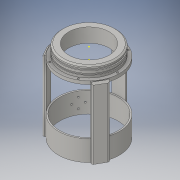
# Autodesk Inventor part: O ring fitting with motor mount
Saved by Autodesk Inventor 2016 (Build 200138000, 138)
## iProperties
Created: 2017-01-20
Part Number: O ring fitting with motor mount
Material: Generic
Document SubType Name: Modeling
Designer: Student
Density: 1 g/cm^3
Appearance: Default
Author: Student
Autodesk Inventor part; units mm, degrees
ref_plane "YZ Plane" through (0, 0, 0) normal (1, 0, 0) x (0, 1, 0)
ref_plane "XZ Plane" through (0, 0, 0) normal (0, 1, 0) x (-1, 0, 0)
ref_plane "XY Plane" through (0, 0, 0) normal (0, 0, 1) x (1, 0, 0)
sketch "Sketch1" plane through (0, 0, 0) normal (0, 1, 0) x (-1, 0, 0)
  circle A0 centre (0, 0) radius 50.8
  dimension "d0" = 101.6
  constraints: 1 centre point, 1 coincident
  measures "d0" diameter of A0
extrude "Extrusion1" add sketch "Sketch1" along normal blind 7.62
sketch "Sketch2" plane through (0, 7.62, 0) normal (0, 1, 0) x (1, 0, 0)
  circle A0 centre (0, 0) radius 49.2125
  circle A1 centre (0, 0) radius 50.8
  dimension "d3" = 98.425
  constraints: 2 centre point, 2 coincident
  measures "d3" diameter of A0
extrude "Extrusion2" cut sketch "Sketch2" against normal blind 3.175
sketch "Sketch3" plane through (0, 7.62, 0) normal (0, 1, 0) x (1, 0, 0)
  circle A0 centre (0, 0) radius 50.9584
  constraints: 1 centre point, 1 coincident
extrude "Extrusion3" add sketch "Sketch3" along normal blind 7.62
sketch "Sketch4" plane through (0, 15.24, 0) normal (0, 1, 0) x (1, 0, 0)
  point P0 (0, 0)
sketch "Sketch5" plane through (0, 15.24, 0) normal (0, 1, 0) x (1, 0, 0)
  circle A0 centre (0, 0) radius 49.2125
  circle A1 centre (0, 0) radius 50.9584
  dimension "d8" = 98.425
  constraints: 2 centre point, 2 coincident
  measures "d8" diameter of A0
extrude "Extrusion4" cut sketch "Sketch5" against normal blind 3.175
sketch "Sketch6" plane through (0, 15.24, 0) normal (0, 1, 0) x (1, 0, 0)
  circle A0 centre (0, 0) radius 50.8
  dimension "d11" = 101.6
  constraints: 1 centre point, 1 coincident
  measures "d11" diameter of A0
extrude "Extrusion5" add sketch "Sketch6" along normal blind 5.08
sketch "Sketch7" plane through (0, 0, 0) normal (0, -1, 0) x (1, 0, 0)
  circle A0 centre (0, 0) radius 57.15
  dimension "d14" = 114.3
  constraints: 1 centre point, 1 coincident
  measures "d14" diameter of A0
extrude "Extrusion6" add sketch "Sketch7" along normal blind 6.096
chamfer "Chamfer1" distance 2.54 angle 45 1 edges at (-50.8, 20.32, 0)
sketch "Sketch8" plane through (0, -6.096, 0) normal (0, -1, 0) x (1, 0, 0)
  circle A0 centre (0, 0) radius 50.8
  circle A1 centre (53.975, 0) radius 1.7526
  circle A2 centre (26.9875, 46.7437) radius 1.7526
  circle A3 centre (-26.9875, 46.7437) radius 1.7526
  circle A4 centre (-53.975, 0) radius 1.7526
  circle A5 centre (-26.9875, -46.7437) radius 1.7526
  circle A6 centre (26.9875, -46.7437) radius 1.7526
  dimension "d20" = 3.5052
  dimension "d21" = 53.975
  dimension "d24" = 360
  constraints: 7 centre point, 1 coincident, 13 other
  measures "d20" diameter of A1
  measures "d21" distance of A0.centre A1.centre
extrude "Extrusion7" cut sketch "Sketch8" against normal blind 6.096 contours A1 | A2 | A3 | A4 | A5 | A6
sketch "Sketch9" plane through (0, -6.096, 0) normal (0, -1, 0) x (1, 0, 0)
  circle A0 centre (0, 0) radius 12.7
  circle A1 centre (0, 0) radius 1.27
  dimension "d28" = 25.4
  dimension "d29" = 2.54
  constraints: 2 centre point, 2 coincident
  measures "d28" diameter of A0
  measures "d29" diameter of A1
extrude "Extrusion8" cut sketch "Sketch9" against normal blind 127 contours A1
sketch "Sketch10" plane through (0, -6.096, 0) normal (0, -1, 0) x (1, 0, 0)
  circle A0 centre (0, 0) radius 1.27 projected
  circle A1 centre (0, 0) radius 38.1
  dimension "d33" = 76.2
  constraints: 1 centre point, 1 coincident
  measures "d33" diameter of A1
extrude "Extrusion9" cut sketch "Sketch10" against normal blind 9.525
sketch "Sketch11" plane through (0, 3.429, 0) normal (0, -1, 0) x (1, 0, 0)
  circle A0 centre (0, 0) radius 12.7
  circle A1 centre (0, 0) radius 1.27
  dimension "d36" = 25.4
  constraints: 2 centre point, 2 coincident
  measures "d36" diameter of A0
extrude "Extrusion10" add sketch "Sketch11" along normal blind 9.525
sketch "Sketch12" plane through (0, 20.32, 0) normal (0, 1, 0) x (1, 0, 0)
  circle A0 centre (0, 0) radius 1.27 projected
  circle A1 centre (0, 0) radius 38.1
  constraints: 1 centre point, 1 coincident
extrude "Extrusion11" cut sketch "Sketch12" against normal blind 508
sketch "Sketch13" plane through (0, -6.096, 0) normal (0, -1, 0) x (1, 0, 0)
  point P0 (0, 0)
sketch "Sketch14" plane through (0, -6.096, 0) normal (0, -1, 0) x (1, 0, 0)
  line L0 (0, -60.96) -> (12.7, -60.96)
  line L1 (0, -60.96) -> (-12.7, -60.96)
  circle A0 centre (0, 0) radius 57.15 projected
  arc A1 (-12.7, -55.721) -> (12.7, -55.721) centre (0, 0) ccw
  line L2 (12.7, -60.96) -> (12.7, -55.721)
  line L3 (-12.7, -60.96) -> (-12.7, -55.721)
  line L4 (52.7929, 30.48) -> (59.1429, 19.4815)
  line L5 (52.7929, 30.48) -> (46.4429, 41.4785)
  line L6 (46.4429, 41.4785) -> (41.9058, 38.859)
  arc A2 (54.6058, 16.862) -> (41.9058, 38.859) centre (0, 0) ccw
  line L7 (59.1429, 19.4815) -> (54.6058, 16.862)
  line L8 (-52.7929, 30.48) -> (-46.4429, 41.4785)
  line L9 (-52.7929, 30.48) -> (-59.1429, 19.4815)
  line L10 (-59.1429, 19.4815) -> (-54.6058, 16.862)
  arc A3 (-41.9058, 38.859) -> (-54.6058, 16.862) centre (0, 0) ccw
  line L11 (-46.4429, 41.4785) -> (-41.9058, 38.859)
  point P0 (0, -57.15)
  point P1 (49.4934, 28.575)
  point P2 (-49.4934, 28.575)
  dimension "d41" = 12.7
  dimension "d42" = 12.7
  dimension "d43" = 3.81
  dimension "d46" = 360
  constraints: 24 end point, 12 point on circle, 3 centre point, 2 coincident, 2 horizontal, 1 concentric, 1 parallel, 35 other
  measures "d41" distance of L0.start L1.end
  measures "d42" distance of L0.start L0.end
  measures "d43" distance from line of L1 A0.start
extrude "Extrusion12" add sketch "Sketch14" along normal blind 127 and the other way blind 5.08 contours L1 L3 A0 L2 L0 | L10 L9 L8 L11 A0 | A0 L6 L5 L4 L7
chamfer "Chamfer2" distance 3.175 angle 45 3 edges at (52.7929, -1.016, 30.48) (0, -1.016, -60.96) (-52.7929, -1.016, 30.48)
fillet "Fillet1" radius 3.175 6 edges at (-59.1429, -68.6435, 19.4815) (-46.4429, -68.6435, 41.4785) (-12.7, -68.6435, -60.96) (12.7, -68.6435, -60.96) (59.1429, -68.6435, 19.4815) (46.4429, -68.6435, 41.4785)
ref_plane "Work Plane1" through (-48.2558, -133.096, 27.8605) normal (-0.5, 0, -0.8660254) x (-0.8660254, 0, 0.5)
sketch "Sketch15" plane through (-48.2558, -133.096, 27.8605) normal (-0.5, 0, -0.8660254) x (-0.8660254, 0, 0.5)
  line L0 (-55.721, 148.3202) -> (-55.721, -8.2891)
  line L1 (1.429, 0) -> (0, 0) projected
  line L2 (1.429, 0) -> (-1.111, 0)
  line L3 (-1.111, 0) -> (-1.111, 38.7858)
  line L4 (-1.111, 38.7858) -> (1.429, 38.7858)
  line L5 (1.429, 38.7858) -> (1.429, 0)
  point P0 (-55.721, 133.096)
  dimension "d58" = 2.54
  dimension "d59" = 38.7858
  constraints: 10 end point, 2 parallel, 1 horizontal, 1 perpendicular, 1 vertical
  measures "d58" distance of L1.start L2.end
  measures "d59" distance of L2.end L3.end
revolve "Revolution1" add sketch "Sketch15" angle 360 about axis through (0, 15.2242, 0) along (0, -1, 0)
ref_plane "Work Plane3" through (-43.4442, -113.7031, -25.0825) normal (0.8660254, 0, 0.5) x (0, 1, 0)
ref_plane "Work Plane2" through (47.2936, -113.7031, 27.305) normal (0.8660254, 0, 0.5) x (0, 1, 0)
sketch "Sketch16" plane through (-43.4442, -113.7031, -25.0825) normal (0.8660254, 0, 0.5) x (0, 1, 0)
  line L0 (19.3929, 41.9058) -> (19.3929, -41.9058) projected
  line L1 (19.3929, 0) -> (-60.7336, 0)
  line L2 (19.3929, 54.6058) -> (-19.3929, 54.6058) projected
  line L3 (0, 54.6058) -> (0, -48.0304)
  line L4 (109.5121, -48.0304) -> (-19.3929, -48.0304) projected
  circle A0 centre (9.398, 0) radius 1.4986
  circle A1 centre (-9.398, 0) radius 1.4986
  circle A2 centre (0, -9.398) radius 1.4986
  circle A3 centre (0, 9.398) radius 1.4986
  point P0 (113.7031, 0)
  dimension "d64" = 2.9972
  dimension "d65" = 2.9972
  dimension "d66" = 2.9972
  dimension "d67" = 2.9972
  dimension "d68" = 18.796
  dimension "d69" = 18.796
  dimension "d70" = 18.796
  dimension "d71" = 18.796
  constraints: 5 point on line, 4 centre point, 4 end point, 2 midpoint, 1 horizontal, 1 vertical
  measures "d64" diameter of A0
  measures "d65" diameter of A2
  measures "d66" diameter of A1
  measures "d67" diameter of A3
  measures "d68" diameter of A2.centre L1
  measures "d69" diameter of A3.centre L1
  measures "d70" diameter of A0.centre L3
  measures "d71" diameter of A1.centre L3
extrude "Extrusion13" cut sketch "Sketch16" against normal blind 127
equation "\"d42\" = d41"
equation "\"d65\" = d64"
equation "\"d66\" = d65"
equation "\"d67\" = d64"
equation "\"d68\" = d69"
equation "\"d71\" = d70"
body "Solid1"
